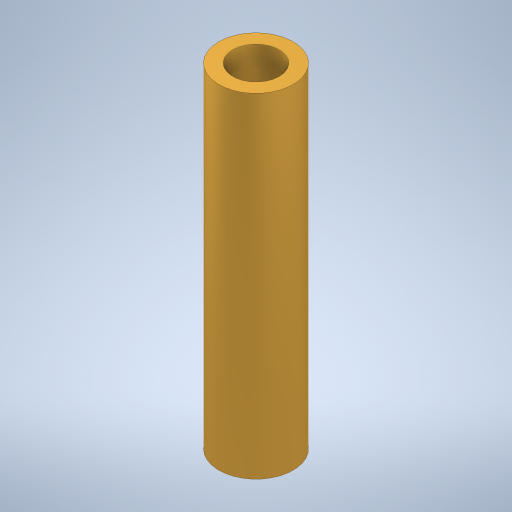
# Autodesk Inventor part: Espaçador do motor
Saved by Autodesk Inventor 2023 (Build 270158000, 158)
## iProperties
Created: 2023-03-21
Part Number: Espaçador do motor
Material: Brass, Soft Yellow
Document SubType Name: Sheet Metal
Designer: Mateus
Density: 8.47 g/cm^3
Sheet Metal Rule: Default_mm
Appearance: Brass - Satin
Mass: 5.77422 g
Surface Area: 14.0743 cm^2
Volume: 0.681726 cm^3
Author: Mateus
Autodesk Inventor part; units mm, degrees
ref_plane "YZ Plane" through (0, 0, 0) normal (1, 0, 0) x (0, 1, 0)
ref_plane "XZ Plane" through (0, 0, 0) normal (0, 1, 0) x (-1, 0, 0)
ref_plane "XY Plane" through (0, 0, 0) normal (0, 0, 1) x (1, 0, 0)
sketch "Esboço1" plane through (0, 0, 0) normal (0, 1, 0) x (-1, 0, 0)
  circle A0 centre (0, 0) radius 4
  dimension "d1" = 8
  constraints: 1 centre point
  measures "d1" diameter of A0
extrude "Extrusão1" add sketch "Esboço1" along normal blind 36
sketch "Esboço2" plane through (0, 36, 0) normal (0, 1, 0) x (1, 0, 0)
  circle A0 centre (0, 0) radius 4 projected
  constraints: 1 coincident
hole "Furo1" at (0, 36, 0) direction (0, -1, 0) diameter 5 end through all
equation "\"d9\" = Espessura"
equation "\"Raio_vergadura\" = Espessura"
equation "\"Largura_alívio_de_vergadura\" = Espessura"
equation "\"Profundidade_alívio_de_vergadura\" = 0.5 * Espessura"
equation "\"Tamanho_alívio_de_dobra\" = 4 * Espessura"
equation "\"Remanescente_mínimo\" = 2 * Espessura"
equation "\"Raiodetransição\" = Raio_vergadura"
equation "\"Tamanho_de_raio_de_Jacobi\" = Raio_vergadura"
equation "\"TamanhoFolga\" = Espessura"
equation "\"Espessura\" = 0.5"
